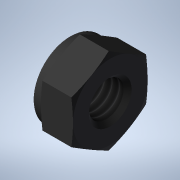
# Autodesk Inventor part: UNUTZ4
Saved by Autodesk Inventor 2021 (Build 250183000, 183)
## iProperties
Created: 2025-11-06
Part Number: UNUTZ4
Material: Generic
Catalog Web Link: www.3dfindit.com
Description: UNUTZ, UNUTKZ, UNUTSZ-U Nut
Vendor: MISUMI
Document SubType Name: Modeling
Designer: psAdmin
Manufacturer: MISUMI
Mass: 0.115356 g
Surface Area: 2.00728 cm^2
Volume: 0.115356 cm^3
Density: 1 g/cm^3
Appearance: PSOLRGB-176-176-176
Category: PARTsolutions
Company: MISUMI
Title: UNUTZ4
Author: Cadenas PARTsolutions
Comments: U Nut
PSOL_IDENT_0: {$CADENAS_DATA/23d-libs/misumi/metric/27_screws_nuts/unutkz.prj},174 {VTYP=3D},{NB=UNUTZ4},{LINA=UNU
PSOL_IDENT_1: TZ4},{NN=UNUTZ, UNUTKZ, UNUTSZ},{DATE=29.11.2024 04:24:51},{GEOMDATE=31.10.2013 09:16:00},{VERSION=}
PSOL_IDENT_2: ,{LINEID=10},{WBVAR=MATB,ST},{WBNUMERIC=}  {NB=UNUTZ4},{LINA=UNUTZ4},{KT=DUMMY},{PN=UNUTZ4},{TYPE=UN
PSOL_IDENT_3: UTZ},{MATB=},{MATFR=SUS301},{ST=B},{ST0='B','Bright Chromate Plating','T','Trivalent Chromate'},{PS=
PSOL_IDENT_4: JIS6H (Class 2)},{M=4},{P=0.70},{SREF=7},{STOL=0/-0.2},{HHREF=3.8},{HHTOL=+0.3/-0.3},{MM=3.0},{EE=8.
PSOL_IDENT_5: 1},{TT=2.2 (22)}
NB: UNUTZ4
NN: UNUTZ, UNUTKZ, UNUTSZ
NT: U Nut
NBSYN: $PN.
LINA: UNUTZ4
CATALOG: Misumi
PN: UNUTZ4
MATB: 1018 Carbon Steel or Equivalent
MATFR: SUS301
ST: Bright Chromate Plating
PS: JIS6H (Class 2)
M: 4
P: 0.7
SREF: 7
STOL: 0/-0.2
HHREF: 3.8
HHTOL: +0.3/-0.3
MM: 3
EE: 8.1
TT: 2.2 (22)
SUPPLIER: MISUMI
ARTICLENO: UNUTZ4
BOMINFO: UNUTZ4
CREATOR: CADENAS GmbH
Autodesk Inventor part; units mm, degrees
sketch "Sketch_1" plane through (0, 0, 0) normal (0, 0, 1) x (1, 0, 0)
  line L0 (1.9, 0) -> (-1.1, 0)
  line L1 (-1.1, 0) -> (-1.1, 2.75)
  line L2 (-1.1, 2.75) -> (-1.9, 2.75)
  line L3 (-1.9, 2.75) -> (-1.9, 3.3)
  arc A0 (-1.7, 3.5) -> (-1.9, 3.3) centre (-1.7, 3.3) ccw
  line L4 (-1.7, 3.5) -> (-1.1, 3.5)
  line L5 (-1.1, 3.5) -> (-0.9526, 4.05)
  line L6 (-0.9526, 4.05) -> (1.7526, 4.05)
  line L7 (1.7526, 4.05) -> (1.9, 3.5)
  line L8 (1.9, 3.5) -> (1.9, 0)
  line L9 (1.9, 0) -> (-1.1, 0)
  constraints: 20 end point, 2 point on circle, 1 centre point
revolve "Revolution1" add sketch "Sketch_1" angle 360 about axis through (1.9, 0, 0) along (1, 0, 0)
sketch "Sketch_2" plane through (0, 0, 0) normal (1, 0, 0) x (0, 1, 0)
  line L0 (7, 7) -> (-7, 7)
  line L1 (-7, 7) -> (-7, -7)
  line L2 (-7, -7) -> (7, -7)
  line L3 (7, -7) -> (7, 7)
  line L4 (-2.0207, 3.5) -> (-4.0415, 0)
  line L5 (-4.0415, 0) -> (-2.0207, -3.5)
  line L6 (-2.0207, -3.5) -> (2.0207, -3.5)
  line L7 (2.0207, -3.5) -> (4.0415, 0)
  line L8 (4.0415, 0) -> (2.0207, 3.5)
  line L9 (2.0207, 3.5) -> (-2.0207, 3.5)
  constraints: 20 end point
extrude "Extrusion1" cut sketch "Sketch_2" along normal mid plane 3.8
sketch "Sketch_3" plane through (0, 0, 0) normal (0, 0, 1) x (1, 0, 0)
  line L0 (1.9, 0) -> (-1.1, 0)
  line L1 (-1.1, 0) -> (-1.1, 2)
  line L2 (-1.1, 2) -> (-0.721, 1.621)
  line L3 (-0.721, 1.621) -> (1.521, 1.621)
  line L4 (1.521, 1.621) -> (1.9, 2)
  line L5 (1.9, 2) -> (1.9, 0)
  line L6 (1.9, 0) -> (-1.1, 0)
  constraints: 14 end point
revolve "Revolution2" cut sketch "Sketch_3" angle 360 about axis through (1.9, 0, 0) along (1, 0, 0)
thread "Thread1" size "M4x0.7" class "6H" standard "ISO Metric profile" full length
sketch "Sketch_7" plane through (-1.1, 0, 0) normal (1, 0, 0) x (0, 0, -1)
  line L0 (-1.375, 2.3816) -> (-0.8, 1.3856)
  arc A0 (0.8, 1.3856) -> (-0.8, 1.3856) centre (0, 0) ccw
  line L1 (0.8, 1.3856) -> (1.375, 2.3816)
  arc A1 (1.375, 2.3816) -> (-1.375, 2.3816) centre (0, 0) ccw
  constraints: 4 end point, 4 point on circle, 2 centre point
extrude "Extrusion2" add sketch "Sketch_7" against normal blind 0.4
sketch "Sketch_9" plane through (-1.1, 0, 0) normal (1, 0, 0) x (0, 0, -1)
  arc A0 (-2.75, 0) -> (-1.375, -2.3816) centre (0, 0) ccw
  line L0 (-1.375, -2.3816) -> (-0.8, -1.3856)
  arc A1 (-1.6, 0) -> (-0.8, -1.3856) centre (0, 0) ccw
  line L1 (-1.6, 0) -> (-2.75, 0)
  constraints: 4 end point, 4 point on circle, 2 centre point
extrude "Extrusion3" add sketch "Sketch_9" against normal blind 0.4
sketch "Sketch_8" plane through (-1.1, 0, 0) normal (1, 0, 0) x (0, 0, -1)
  line L0 (0.8, -1.3856) -> (1.375, -2.3816)
  arc A0 (1.375, -2.3816) -> (2.75, 0) centre (0, 0) ccw
  line L1 (2.75, 0) -> (1.6, 0)
  arc A1 (0.8, -1.3856) -> (1.6, 0) centre (0, 0) ccw
  constraints: 4 end point, 4 point on circle, 2 centre point
extrude "Extrusion4" add sketch "Sketch_8" against normal blind 0.4
ref_plane "to_bolt_XY" through (1.9, 0, 0) normal (1, 0, 0) x (0, 0, -1)
ref_plane "to_bolt_YZ" through (1.9, 0, 0) normal (0, 0, -1) x (0, 1, 0)
ref_plane "to_bolt_ZX" through (1.9, 0, 0) normal (0, 1, 0) x (1, 0, 0)
body "Solid1"
